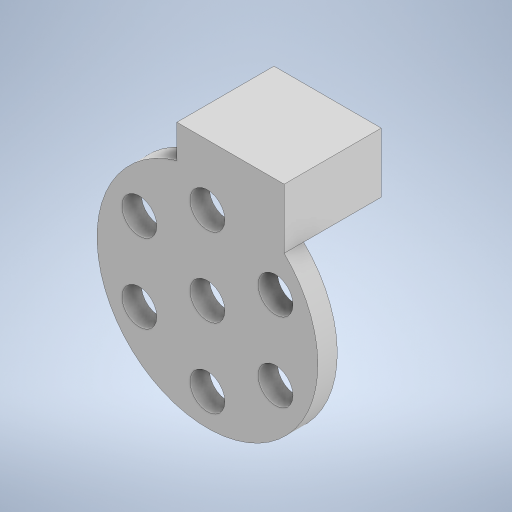
# Autodesk Inventor part: revolver
Saved by Autodesk Inventor 2023.1 (Build 271208000, 208)
## iProperties
Created: 2023-04-12
Part Number: revolver
Material: Типовые
Document SubType Name: Modeling
Designer: User
Density: 1 g/cm^3
Appearance: По умолчанию
Author: User
Autodesk Inventor part; units mm, degrees
(part 1 of 8)
ref_plane "YZ Plane" through (0, 0, 0) normal (1, 0, 0) x (0, 1, 0)
ref_plane "XZ Plane" through (0, 0, 0) normal (0, 1, 0) x (-1, 0, 0)
ref_plane "XY Plane" through (0, 0, 0) normal (0, 0, 1) x (1, 0, 0)
sketch "Эскиз1" plane through (0, 0, 0) normal (0, 0, 1) x (1, 0, 0)
  line L0 (-22.838, -17.5712) -> (24.4153, -17.5965)
  arc A0 (24.4153, -17.5965) -> (25.2491, -16.7631) centre (24.4158, -16.7631) ccw
  line L1 (25.2491, -16.7631) -> (25.2491, 45.1296)
  arc A1 (25.2491, 45.1296) -> (24.4158, 45.963) centre (24.4158, 45.1296) ccw
  line L2 (24.4158, 45.963) -> (-5.7821, 45.963)
  line L3 (-5.7821, 45.963) -> (-5.7821, 46.7963)
  line L4 (-5.7821, 46.7963) -> (24.4158, 46.7963)
  arc A2 (26.0825, 45.1296) -> (24.4158, 46.7963) centre (24.4158, 45.1296) ccw
  line L5 (26.0825, 45.1296) -> (26.0825, -16.7631)
  arc A3 (24.4149, -18.4298) -> (26.0825, -16.7631) centre (24.4158, -16.7631) ccw
  line L6 (24.4149, -18.4298) -> (-22.851, -18.4045)
  arc A4 (-24.5167, -16.7369) -> (-22.851, -18.4045) centre (-22.8501, -16.7378) ccw
  line L7 (-24.5167, -16.7369) -> (-24.5023, 10.1628)
  line L8 (-24.5023, 10.1628) -> (-24.5023, 45.1296)
  arc A5 (-22.8357, 46.7963) -> (-24.5023, 45.1296) centre (-22.8357, 45.1296) ccw
  line L9 (-22.8357, 46.7963) -> (-21.4453, 46.7963)
  line L10 (-21.4453, 46.7963) -> (-21.4453, 45.9649)
  line L11 (-21.4453, 45.9649) -> (-22.8357, 45.9649)
  arc A6 (-22.8357, 45.9649) -> (-23.6709, 45.1296) centre (-22.8357, 45.1296) ccw
  line L12 (-23.6709, 45.1296) -> (-23.6709, -16.7378)
  arc A7 (-23.6709, -16.7378) -> (-22.838, -17.5712) centre (-22.8376, -16.7378) ccw
  arc A8 (-21.1689, 72.3508) -> (-19.5022, 70.6842) centre (-19.5022, 72.3508) ccw
  line L13 (-21.1689, 72.3508) -> (-21.1689, 75.1651)
  arc A9 (-19.5022, 76.8318) -> (-21.1689, 75.1651) centre (-19.5022, 75.1651) ccw
  line L14 (-19.5022, 76.8318) -> (21.0482, 76.8318)
  arc A10 (22.7149, 75.1651) -> (21.0482, 76.8318) centre (21.0482, 75.1651) ccw
  line L15 (22.7149, 75.1651) -> (22.7149, 72.3508)
  arc A11 (21.0482, 70.6842) -> (22.7149, 72.3508) centre (21.0482, 72.3508) ccw
  line L16 (21.0482, 70.6842) -> (-19.5022, 70.6842)
  arc A12 (-21.1685, 54.6279) -> (-19.5018, 52.9613) centre (-19.5018, 54.6279) ccw
  line L17 (-21.1685, 54.6279) -> (-21.1685, 67.6609)
  arc A13 (-19.5018, 69.3275) -> (-21.1685, 67.6609) centre (-19.5018, 67.6609) ccw
  line L18 (-19.5018, 69.3275) -> (21.0483, 69.3275)
  arc A14 (22.715, 67.6609) -> (21.0483, 69.3275) centre (21.0483, 67.6609) ccw
  line L19 (22.715, 67.6609) -> (22.715, 54.6279)
  arc A15 (21.0483, 52.9613) -> (22.715, 54.6279) centre (21.0483, 54.6279) ccw
  line L20 (21.0483, 52.9613) -> (-19.5018, 52.9613)
  line L21 (19.3067, -63.6373) -> (19.3067, -61.3545)
  line L22 (19.3067, -61.3545) -> (18.828, -61.3545)
  line L23 (18.828, -61.3545) -> (18.0508, -63.7032)
  line L24 (7.2647, -61.3545) -> (6.4355, -61.3545)
  line L25 (6.4355, -61.3545) -> (6.4355, -63.6373)
  line L26 (4.7702, -63.0128) -> (4.7702, -61.3545)
  line L27 (4.7702, -61.3545) -> (3.9411, -61.3545)
  line L28 (-4.7774, -61.1463) -> (-4.7774, -62.1837)
  line L29 (-4.7774, -62.1837) -> (-3.5353, -62.1837)
  line L30 (-3.5353, -62.1837) -> (-3.5353, -61.1463)
  line L31 (-3.5353, -63.6373) -> (-3.5353, -62.6)
  line L32 (-3.5353, -62.6) -> (-4.7774, -62.6)
  line L33 (-4.7774, -62.6) -> (-4.7774, -63.6373)
  line L34 (-13.5409, -61.1463) -> (-13.5409, -62.371)
  line L35 (-13.5409, -62.371) -> (-12.2225, -60.9868)
  line L36 (-11.9485, -61.3025) -> (-12.7846, -62.1802)
  line L37 (-12.7846, -62.1802) -> (-11.9276, -63.502)
  line L38 (-15.1645, -63.0128) -> (-15.1645, -61.3545)
  line L39 (-15.1645, -61.3545) -> (-15.9937, -61.3545)
  line L40 (-10.0766, -55.8058) -> (-10.8765, -54.608)
  line L41 (-10.8765, -54.608) -> (-11.6765, -55.8058)
  line L42 (-12.104, -55.5222) -> (-11.1855, -54.1466)
  line L43 (-11.1855, -54.1466) -> (-12.104, -52.771)
  line L44 (-11.6765, -52.4875) -> (-10.8765, -53.6853)
  line L45 (-10.8765, -53.6853) -> (-10.0766, -52.4875)
  line L46 (-9.6491, -52.771) -> (-10.5676, -54.1466)
  line L47 (-10.5676, -54.1466) -> (-9.6491, -55.5222)
  line L48 (-20.3629, -49.5032) -> (-18.6809, -54.4768)
  line L49 (-18.6809, -54.4768) -> (-16.999, -49.5032)
  line L50 (14.3835, -41.5364) -> (15.2126, -41.5364)
  line L51 (15.2126, -41.5364) -> (15.2126, -40.7072)
  line L52 (15.2126, -40.7072) -> (14.3835, -40.7072)
  line L53 (15.2126, -42.99) -> (15.2126, -41.9527)
  line L54 (15.2126, -41.9527) -> (14.7026, -41.9527)
  line L55 (14.7026, -41.9527) -> (13.9359, -43.1045)
  line L56 (12.3053, -42.3655) -> (12.3053, -40.7072)
  line L57 (12.3053, -40.7072) -> (11.4762, -40.7072)
  line L58 (-0.9857, -42.99) -> (-0.9857, -40.7072)
  line L59 (-0.9857, -40.7072) -> (-1.4645, -40.7072)
  line L60 (-1.4645, -40.7072) -> (-2.2416, -43.0559)
  line L61 (-13.0277, -40.7072) -> (-13.8569, -40.7072)
  line L62 (-13.8569, -40.7072) -> (-13.8569, -42.99)
  line L63 (-15.5222, -42.3655) -> (-15.5222, -40.7072)
  line L64 (-15.5222, -40.7072) -> (-16.3514, -40.7072)
  line L65 (20.5386, -19.6576) -> (19.7094, -19.6576)
  line L66 (19.7094, -19.6576) -> (19.7094, -21.7323)
  line L67 (19.7094, -21.7323) -> (20.5386, -21.7323)
  line L68 (20.5386, -22.1486) -> (19.7094, -22.1486)
  line L69 (19.7094, -22.1486) -> (19.7094, -23.186)
  line L70 (16.8021, -20.0705) -> (16.8021, -20.4868)
  line L71 (16.8021, -20.4868) -> (18.0442, -20.4868)
  line L72 (18.0442, -20.4868) -> (18.0442, -20.0705)
  line L73 (18.2523, -20.9031) -> (16.8021, -20.9031)
  line L74 (16.8021, -20.9031) -> (16.8021, -21.316)
  line L75 (-18.1801, -30.8646) -> (-18.1801, -34.3929)
  line L76 (-18.1801, -34.3929) -> (-16.7265, -34.3929)
  line L77 (-6.2745, -20.9508) -> (-7.1037, -20.9508)
  line L78 (-7.1037, -20.9508) -> (-7.1037, -21.78)
  line L79 (-7.1037, -21.78) -> (-6.2745, -21.78)
  line L80 (-7.1037, -19.4972) -> (-7.1037, -20.5345)
  line L81 (-7.1037, -20.5345) -> (-6.2745, -20.5345)
  line L82 (-12.0891, -21.78) -> (-11.26, -21.78)
  line L83 (-11.26, -21.78) -> (-11.26, -19.4972)
  line L84 (8.677, -7.6777) -> (7.8478, -7.6777)
  line L85 (7.8478, -7.6777) -> (7.8478, -9.9605)
  line L86 (6.1825, -9.336) -> (6.1825, -7.6777)
  line L87 (6.1825, -7.6777) -> (5.3534, -7.6777)
  line L88 (6.8528, 0.8169) -> (6.0236, 0.8169)
  line L89 (6.0236, 0.8169) -> (6.0236, -1.4659)
  line L90 (-11.1301, -10.0439) -> (-11.1301, -9.2147)
  line L91 (-11.1301, -9.2147) -> (-12.3756, -9.2147)
  line L92 (-12.3722, -8.7984) -> (-11.1301, -8.7984)
  line L93 (-11.1301, -8.7984) -> (-11.1301, -6.9319)
  line L94 (-17.146, -7.1401) -> (-18.6031, -7.1401)
  line L95 (-18.6031, -7.1401) -> (-18.6031, -8.3856)
  line L96 (-18.6031, -8.3856) -> (-17.5588, -8.3856)
  line L97 (-17.5588, -8.8019) -> (-18.6031, -8.8019)
  line L98 (-18.6031, -8.8019) -> (-18.6031, -10.4602)
  line L99 (-18.6031, -10.4602) -> (-17.146, -10.4602)
  line L100 (-8.8573, 0.7006) -> (-9.6865, 0.7006)
  line L101 (-9.6865, 0.7006) -> (-9.6865, -1.3741)
  line L102 (-9.6865, -1.3741) -> (-8.8573, -1.3741)
  line L103 (-8.8573, -1.7904) -> (-9.6865, -1.7904)
  line L104 (-9.6865, -1.7904) -> (-9.6865, -2.8277)
  line L105 (-18.4084, 0.9087) -> (-18.4084, -0.1286)
  line L106 (-18.4084, -0.1286) -> (-17.1664, -0.1286)
  line L107 (-17.1664, -0.1286) -> (-17.1664, 0.9087)
  line L108 (-17.1664, -1.5823) -> (-17.1664, -0.5449)
  line L109 (-17.1664, -0.5449) -> (-18.4084, -0.5449)
  line L110 (-18.4084, -0.5449) -> (-18.4084, -1.5823)
  line L111 (17.3177, 22.7837) -> (17.3177, 24.5136)
  line L112 (17.3177, 24.5136) -> (16.7676, 24.5136)
  line L113 (16.7676, 24.5136) -> (16.7676, 22.7837)
  line L114 (18.0107, 24.5136) -> (17.7357, 24.5136)
  line L115 (17.7357, 24.5136) -> (17.7357, 22.7837)
  line L116 (12.8402, 24.5136) -> (12.2407, 24.5136)
  line L117 (12.2407, 24.5136) -> (12.2407, 22.7837)
  line L118 (-7.5678, 13.3431) -> (-7.5678, 16.3093)
  line L119 (-7.5678, 16.3093) -> (-8.4247, 14.873)
  line L120 (-8.782, 14.873) -> (-9.6459, 16.3093)
  line L121 (-9.6459, 16.3093) -> (-9.6459, 13.3431)
  line L122 (-9.6737, 17.1697) -> (-8.6051, 15.3865)
  line L123 (-8.6051, 15.3865) -> (-7.54, 17.1697)
  line L124 (-15.6721, 13.5512) -> (-14.6348, 13.5512)
  line L125 (-14.6348, 13.5512) -> (-14.6348, 15.2096)
  line L126 (-14.6348, 15.2096) -> (-14.8395, 15.2096)
  line L127 (-15.6588, 18.5916) -> (-14.6215, 18.5916)
  line L128 (-14.6215, 18.5916) -> (-14.6215, 20.2499)
  line L129 (-14.6215, 20.2499) -> (-14.8262, 20.2499)
  line L130 (-14.5012, 31.7916) -> (-13.0071, 31.7916)
  line L131 (-13.0071, 31.7916) -> (-13.7521, 34.0264)
  line L132 (-13.7521, 34.0264) -> (-14.5012, 31.7916)
  line L133 (-12.4696, 30.179) -> (-12.8336, 31.2752)
  line L134 (-12.8336, 31.2752) -> (-14.6748, 31.2752)
  line L135 (-14.6748, 31.2752) -> (-15.0388, 30.179)
  line L136 (-18.0947, 32.5323) -> (-19.1063, 32.5323)
  line L137 (-19.1063, 32.5323) -> (-19.1063, 30.5091)
  line L138 (-19.1063, 30.5091) -> (-18.0947, 30.5091)
  line L139 (-17.0831, 34.5597) -> (-19.1063, 34.5597)
  line L140 (-19.1063, 34.5597) -> (-19.1063, 33.0402)
  line L141 (-19.1063, 33.0402) -> (-18.0947, 33.0402)
  line L142 (12.3369, 89.0704) -> (15.2204, 89.0704)
  line L143 (15.2204, 89.0704) -> (15.2204, 84.693)
  line L144 (15.2204, 84.693) -> (14.483, 84.693)
  line L145 (14.483, 84.693) -> (14.483, 88.4511)
  line L146 (14.483, 88.4511) -> (12.9798, 88.4511)
  line L147 (11.3583, 84.693) -> (11.3583, 85.3359)
  line L148 (11.3583, 85.3359) -> (11.3961, 85.3359)
  line L149 (3.7854, 84.9152) -> (3.7854, 83.0811)
  line L150 (3.7854, 83.0811) -> (3.048, 83.0811)
  line L151 (3.048, 83.0811) -> (3.048, 89.0704)
  line L152 (3.048, 89.0704) -> (3.7854, 89.0704)
  line L153 (3.7854, 89.0704) -> (3.7854, 88.6119)
  line L154 (-2.497, 84.693) -> (-2.497, 86.6643)
  line L155 (-2.497, 86.6643) -> (-4.473, 86.6643)
  line L156 (-4.473, 86.6643) -> (-4.473, 84.693)
  line L157 (-4.473, 84.693) -> (-5.2104, 84.693)
  line L158 (-5.2104, 84.693) -> (-5.2104, 89.0704)
  line L159 (-5.2104, 89.0704) -> (-4.473, 89.0704)
  line L160 (-4.473, 89.0704) -> (-4.473, 87.2977)
  line L161 (-4.473, 87.2977) -> (-2.497, 87.2977)
  line L162 (-2.497, 87.2977) -> (-2.497, 89.0704)
  line L163 (-2.497, 89.0704) -> (-1.7596, 89.0704)
  line L164 (-1.7596, 89.0704) -> (-1.7596, 84.693)
  line L165 (-1.7596, 84.693) -> (-2.497, 84.693)
  line L166 (-1.6305, 80.6448) -> (-2.0468, 80.6448)
  line L167 (-2.0468, 80.6448) -> (-2.0468, 79.8157)
  line L168 (-2.0468, 79.8157) -> (-1.6305, 79.8157)
  line L169 (-2.0468, 82.0985) -> (-2.0468, 81.0612)
  line L170 (-2.0468, 81.0612) -> (-1.6305, 81.0612)
  line L171 (-11.1885, 79.6075) -> (-11.1885, 81.8903)
  line L172 (-11.1885, 81.8903) -> (-12.0177, 81.8903)
  line L173 (-12.0177, 81.8903) -> (-12.0177, 79.6075)
  line L174 (-10.3559, 81.8903) -> (-10.7722, 81.8903)
  line L175 (-10.7722, 81.8903) -> (-10.7722, 79.6075)
  line L176 (-17.0031, 79.8157) -> (-16.174, 79.8157)
  line L177 (-16.174, 79.8157) -> (-16.174, 82.0985)
  arc A16 (-22.8351, -20.4439) -> (-24.5018, -22.1106) centre (-22.8351, -22.1106) ccw
  line L178 (-22.8351, -20.4439) -> (-21.4448, -20.4439)
  line L179 (-21.4448, -20.4439) -> (-21.4448, -21.2772)
  line L180 (-21.4448, -21.2772) -> (-22.8351, -21.2772)
  arc A17 (-22.8351, -21.2772) -> (-23.6685, -22.1106) centre (-22.8351, -22.1106) ccw
  line L181 (-23.6685, -22.1106) -> (-23.6685, -35.3124)
  arc A18 (-23.6685, -35.3124) -> (-22.8351, -36.1457) centre (-22.8351, -35.3124) ccw
  line L182 (-22.8351, -36.1457) -> (-0.1596, -36.1457)
  arc A19 (-0.1596, -36.1457) -> (0.6737, -35.3124) centre (-0.1596, -35.3124) ccw
  line L183 (0.6737, -35.3124) -> (0.6737, -22.1106)
  arc A20 (0.6737, -22.1106) -> (-0.1596, -21.2772) centre (-0.1596, -22.1106) ccw
  line L184 (-0.1596, -21.2772) -> (-2.846, -21.2772)
  line L185 (-2.846, -21.2772) -> (-2.846, -20.4439)
  line L186 (-2.846, -20.4439) -> (-0.1596, -20.4439)
  arc A21 (1.5071, -22.1106) -> (-0.1596, -20.4439) centre (-0.1596, -22.1106) ccw
  line L187 (1.5071, -22.1106) -> (1.5071, -35.3124)
  arc A22 (-0.1596, -36.9791) -> (1.5071, -35.3124) centre (-0.1596, -35.3124) ccw
  line L188 (-0.1596, -36.9791) -> (-22.8351, -36.9791)
  arc A23 (-24.5018, -35.3124) -> (-22.8351, -36.9791) centre (-22.8351, -35.3124) ccw
  line L189 (-24.5018, -35.3124) -> (-24.5018, -22.1106)
  line L190 (5.6148, -20.4439) -> (5.6148, -21.2772)
  line L191 (5.6148, -21.2772) -> (4.9165, -21.2772)
  arc A24 (4.9165, -21.2772) -> (4.0832, -22.1106) centre (4.9165, -22.1106) ccw
  line L192 (4.0832, -22.1106) -> (4.0832, -35.3124)
  arc A25 (4.0832, -35.3124) -> (4.9165, -36.1457) centre (4.9165, -35.3124) ccw
  line L193 (4.9165, -36.1457) -> (24.3817, -36.1457)
  arc A26 (24.3817, -36.1457) -> (25.215, -35.3124) centre (24.3817, -35.3124) ccw
  line L194 (25.215, -35.3124) -> (25.215, -22.1106)
  arc A27 (25.215, -22.1106) -> (24.3817, -21.2772) centre (24.3817, -22.1106) ccw
  line L195 (24.3817, -21.2772) -> (23.3418, -21.2772)
  line L196 (23.3418, -21.2772) -> (23.3418, -20.4439)
  line L197 (23.3418, -20.4439) -> (24.3817, -20.4439)
  arc A28 (26.0483, -22.1106) -> (24.3817, -20.4439) centre (24.3817, -22.1106) ccw
  line L198 (26.0483, -22.1106) -> (26.0483, -35.3124)
  arc A29 (24.3817, -36.9791) -> (26.0483, -35.3124) centre (24.3817, -35.3124) ccw
  line L199 (24.3817, -36.9791) -> (4.9165, -36.9791)
  arc A30 (3.2498, -35.3124) -> (4.9165, -36.9791) centre (4.9165, -35.3124) ccw
  line L200 (3.2498, -35.3124) -> (3.2498, -22.1106)
  arc A31 (4.9165, -20.4439) -> (3.2498, -22.1106) centre (4.9165, -22.1106) ccw
  line L201 (4.9165, -20.4439) -> (5.6148, -20.4439)
  arc A32 (-22.9167, -41.4487) -> (-24.5833, -43.1153) centre (-22.9167, -43.1153) ccw
  line L202 (-22.9167, -41.4487) -> (-21.4448, -41.4487)
  line L203 (-21.4448, -41.4487) -> (-21.4448, -42.282)
  line L204 (-21.4448, -42.282) -> (-22.9167, -42.282)
  arc A33 (-22.9167, -42.282) -> (-23.75, -43.1153) centre (-22.9167, -43.1153) ccw
  line L205 (-23.75, -43.1153) -> (-23.75, -85.5941)
  arc A34 (-23.75, -85.5941) -> (-22.9167, -86.4275) centre (-22.9167, -85.5941) ccw
  line L206 (-22.9167, -86.4275) -> (24.1667, -86.4275)
  arc A35 (24.1667, -86.4275) -> (25, -85.5941) centre (24.1667, -85.5941) ccw
  line L207 (25, -85.5941) -> (25, -43.1153)
  arc A36 (25, -43.1153) -> (24.1667, -42.282) centre (24.1667, -43.1153) ccw
  line L208 (24.1667, -42.282) -> (17.2706, -42.282)
  line L209 (17.2706, -42.282) -> (17.2706, -41.4487)
  line L210 (17.2706, -41.4487) -> (24.1667, -41.4487)
  arc A37 (25.8333, -43.1153) -> (24.1667, -41.4487) centre (24.1667, -43.1153) ccw
  line L211 (25.8333, -43.1153) -> (25.8333, -85.5941)
  arc A38 (24.1667, -87.2608) -> (25.8333, -85.5941) centre (24.1667, -85.5941) ccw
  line L212 (24.1667, -87.2608) -> (-22.9167, -87.2608)
  arc A39 (-24.5833, -85.5941) -> (-22.9167, -87.2608) centre (-22.9167, -85.5941) ccw
  line L213 (-24.5833, -85.5941) -> (-24.5833, -43.1153)
  line L214 (-8.2778, 81.4775) -> (-8.2778, 81.0612)
  line L215 (-8.2778, 81.0612) -> (-7.0357, 81.0612)
  line L216 (-7.0357, 81.0612) -> (-7.0357, 81.4775)
  line L217 (-6.8276, 80.6448) -> (-8.2778, 80.6448)
  line L218 (-8.2778, 80.6448) -> (-8.2778, 80.232)
  line L219 (-3.7121, 79.6075) -> (-3.7121, 81.4532)
  line L220 (-3.7121, 81.4532) -> (-4.3713, 80.5269)
  line L221 (-4.7113, 80.5269) -> (-5.3705, 81.4532)
  line L222 (-5.3705, 81.4532) -> (-5.3705, 79.6075)
  line L223 (-5.4086, 82.2199) -> (-4.5413, 81.0022)
  line L224 (-4.5413, 81.0022) -> (-3.674, 82.2199)
  line L225 (-11.819, 87.0188) -> (-10.0416, 84.693)
  line L226 (-10.0416, 84.693) -> (-10.9587, 84.693)
  line L227 (-10.9587, 84.693) -> (-12.4572, 86.7115)
  line L228 (-12.4572, 86.7115) -> (-12.8212, 86.7115)
  line L229 (-12.8212, 86.7115) -> (-12.8212, 84.693)
  line L230 (-12.8212, 84.693) -> (-13.5586, 84.693)
  line L231 (-13.5586, 84.693) -> (-13.5586, 89.0704)
  line L232 (-13.5586, 89.0704) -> (-12.8212, 89.0704)
  line L233 (-12.8212, 89.0704) -> (-12.8212, 87.1653)
  line L234 (-10.5427, 89.0704) -> (-10.3441, 89.0704)
  line L235 (-10.3441, 89.0704) -> (-10.3441, 88.4369)
  line L236 (-10.3441, 88.4369) -> (-10.5143, 88.4369)
  line L237 (1.0105, 88.4275) -> (1.0105, 84.693)
  line L238 (1.0105, 84.693) -> (0.2731, 84.693)
  line L239 (0.2731, 84.693) -> (0.2731, 88.4275)
  line L240 (0.2731, 88.4275) -> (-1.216, 88.4275)
  line L241 (-1.216, 88.4275) -> (-1.216, 89.0704)
  line L242 (-1.216, 89.0704) -> (2.4996, 89.0704)
  line L243 (2.4996, 89.0704) -> (2.4996, 88.4275)
  line L244 (2.4996, 88.4275) -> (1.0105, 88.4275)
  line L245 (17.5746, 86.7683) -> (17.0262, 86.7683)
  line L246 (17.0262, 86.7683) -> (17.0262, 85.2792)
  line L247 (17.0262, 85.2792) -> (17.5557, 85.2792)
  line L248 (17.8204, 84.693) -> (16.2888, 84.693)
  line L249 (16.2888, 84.693) -> (16.2888, 89.0704)
  line L250 (16.2888, 89.0704) -> (17.0262, 89.0704)
  line L251 (17.0262, 89.0704) -> (17.0262, 87.3639)
  line L252 (17.0262, 87.3639) -> (17.8393, 87.3639)
  line L253 (-16.8523, 43.0002) -> (-17.6815, 43.0002)
  line L254 (-17.6815, 43.0002) -> (-17.6815, 41.3419)
  line L255 (-17.6815, 41.3419) -> (-16.8523, 41.3419)
  line L256 (-16.8523, 40.9256) -> (-17.6815, 40.9256)
  line L257 (-17.6815, 40.9256) -> (-17.6815, 39.4719)
  line L258 (-14.3579, 43.2084) -> (-14.3579, 41.7548)
  line L259 (-14.3579, 41.7548) -> (-12.6996, 41.7548)
  line L260 (-12.6996, 41.7548) -> (-12.6996, 43.2188)
  line L261 (-12.6996, 39.4719) -> (-12.6996, 41.3384)
  line L262 (-12.6996, 41.3384) -> (-14.3579, 41.3384)
  line L263 (-14.3579, 41.3384) -> (-14.3579, 39.4719)
  line L264 (-4.9187, 31.017) -> (-4.9187, 32.0286)
  line L265 (-4.9187, 32.0286) -> (-6.4382, 32.0286)
  line L266 (-6.4339, 32.5365) -> (-4.9187, 32.5365)
  line L267 (-4.9187, 32.5365) -> (-4.9187, 34.8136)
  line L268 (-12.1271, 21.9117) -> (-12.9562, 21.9117)
  line L269 (-12.9562, 21.9117) -> (-12.9562, 20.2534)
  line L270 (-12.9562, 20.2534) -> (-12.1271, 20.2534)
  line L271 (-12.1271, 19.837) -> (-12.9562, 19.837)
  line L272 (-12.9562, 19.837) -> (-12.9562, 18.3834)
  line L273 (-2.041, 24.5306) -> (-2.6405, 24.5306)
  line L274 (-2.6405, 24.5306) -> (-2.6405, 23.007)
  line L275 (-2.6405, 23.007) -> (-2.041, 23.007)
  line L276 (-2.041, 22.5917) -> (-2.6405, 22.5917)
  line L277 (-2.6405, 22.5917) -> (-2.6405, 21.8326)
  line L278 (0.5003, 23.2848) -> (0.5003, 24.5306)
  line L279 (0.5003, 24.5306) -> (-0.102, 24.5306)
  line L280 (2.1614, 24.9459) -> (2.2412, 24.9459)
  line L281 (2.2412, 24.9459) -> (1.5289, 25.5565)
  line L282 (2.97, 25.4987) -> (2.1312, 25.4987)
  line L283 (2.1312, 25.4987) -> (2.97, 24.7644)
  line L284 (15.3815, 22.2997) -> (15.3815, 22.5747)
  line L285 (15.3815, 22.5747) -> (14.7819, 22.5747)
  line L286 (14.7792, 22.99) -> (15.3815, 22.99)
  line L287 (15.3815, 22.99) -> (15.3815, 24.7199)
  line L288 (-14.2591, -0.9578) -> (-14.2591, 0.7006)
  line L289 (-14.2591, 0.7006) -> (-15.0883, 0.7006)
  line L290 (-11.7646, 0.7006) -> (-12.5938, 0.7006)
  line L291 (-12.5938, 0.7006) -> (-12.5938, -1.5823)
  line L292 (-13.2735, 3.7618) -> (-14.4913, 5.9301)
  line L293 (-14.4913, 5.9301) -> (-14.9839, 5.4444)
  line L294 (-14.9839, 5.4444) -> (-14.9839, 3.8624)
  line L295 (-14.9839, 7.5989) -> (-14.9839, 6.0099)
  line L296 (-14.9839, 6.0099) -> (-13.2354, 7.7446)
  line L297 (-12.9439, 7.4531) -> (-14.1825, 6.2215)
  line L298 (-14.1825, 6.2215) -> (-12.9058, 3.963)
  line L299 (-7.8065, -10.6684) -> (-7.8065, -7.1401)
  line L300 (-7.8065, -7.1401) -> (-9.4649, -7.1401)
  line L301 (-9.4649, -7.1401) -> (-9.4649, -10.6684)
  line L302 (10.1729, -0.8414) -> (10.1729, 0.8169)
  line L303 (10.1729, 0.8169) -> (9.3438, 0.8169)
  line L304 (12.6674, 0.8169) -> (11.8382, 0.8169)
  line L305 (11.8382, 0.8169) -> (11.8382, -1.2577)
  line L306 (11.8382, -1.2577) -> (12.6674, -1.2577)
  line L307 (12.6674, -1.674) -> (11.8382, -1.674)
  line L308 (11.8382, -1.674) -> (11.8382, -2.7114)
  line L309 (11.9971, -9.336) -> (11.9971, -7.6777)
  line L310 (11.9971, -7.6777) -> (11.168, -7.6777)
  line L311 (14.9044, -9.9605) -> (14.9044, -7.6777)
  line L312 (14.9044, -7.6777) -> (14.4257, -7.6777)
  line L313 (14.4257, -7.6777) -> (13.6485, -10.0264)
  line L314 (-17.0746, -21.3637) -> (-17.0746, -19.7053)
  line L315 (-17.0746, -19.7053) -> (-17.9037, -19.7053)
  line L316 (-14.5801, -19.7053) -> (-15.4093, -19.7053)
  line L317 (-15.4093, -19.7053) -> (-15.4093, -21.9882)
  line L318 (-17.474, -25.5939) -> (-18.5114, -25.5939)
  line L319 (-18.5114, -25.5939) -> (-18.5114, -28.914)
  line L320 (-18.5114, -28.914) -> (-17.474, -28.914)
  line L321 (-19.6338, -31.0727) -> (-21.0874, -31.0727)
  line L322 (-21.0874, -31.0727) -> (-21.0874, -32.3113)
  line L323 (-21.0874, -32.3113) -> (-19.6338, -32.3113)
  line L324 (-19.6338, -32.7276) -> (-21.0874, -32.7276)
  line L325 (-21.0874, -32.7276) -> (-21.0874, -34.601)
  line L326 (8.2849, -21.7323) -> (9.1141, -21.7323)
  line L327 (9.1141, -21.7323) -> (9.1141, -19.4495)
  line L328 (15.1369, -21.9405) -> (15.1369, -20.0948)
  line L329 (15.1369, -20.0948) -> (14.4777, -21.0211)
  line L330 (14.1377, -21.0211) -> (13.4785, -20.0948)
  line L331 (13.4785, -20.0948) -> (13.4785, -21.9405)
  line L332 (13.4404, -19.3281) -> (14.3077, -20.5458)
  line L333 (14.3077, -20.5458) -> (15.175, -19.3281)
  line L334 (6.2997, -24.2855) -> (6.4627, -24.2855)
  line L335 (6.4627, -24.2855) -> (5.5329, -23.3973)
  line L336 (7.337, -23.4563) -> (6.1956, -23.4563)
  line L337 (6.1956, -23.4563) -> (7.2954, -24.5075)
  line L338 (10.0361, -26.3601) -> (10.0361, -24.7018)
  line L339 (10.0361, -24.7018) -> (9.207, -24.7018)
  line L340 (12.5306, -24.7018) -> (11.7014, -24.7018)
  line L341 (11.7014, -24.7018) -> (11.7014, -26.7765)
  line L342 (11.7014, -26.7765) -> (12.5306, -26.7765)
  line L343 (12.5306, -27.1928) -> (11.7014, -27.1928)
  line L344 (11.7014, -27.1928) -> (11.7014, -28.2301)
  line L345 (7.0741, -32.5952) -> (7.0741, -30.9369)
  line L346 (7.0741, -30.9369) -> (6.245, -30.9369)
  line L347 (8.6978, -30.7287) -> (8.6978, -31.9534)
  line L348 (8.6978, -31.9534) -> (10.0161, -30.5691)
  line L349 (10.2902, -30.8848) -> (9.4541, -31.7626)
  line L350 (9.4541, -31.7626) -> (10.311, -33.0844)
  line L351 (-19.6715, -40.499) -> (-19.6715, -41.5364)
  line L352 (-19.6715, -41.5364) -> (-18.4295, -41.5364)
  line L353 (-18.4295, -41.5364) -> (-18.4295, -40.499)
  line L354 (-18.4295, -42.99) -> (-18.4295, -41.9527)
  line L355 (-18.4295, -41.9527) -> (-19.6715, -41.9527)
  line L356 (-19.6715, -41.9527) -> (-19.6715, -42.99)
  line L357 (-10.1204, -40.7072) -> (-10.9496, -40.7072)
  line L358 (-10.9496, -40.7072) -> (-10.9496, -42.7819)
  line L359 (-10.9496, -42.7819) -> (-10.1204, -42.7819)
  line L360 (-10.1204, -43.1982) -> (-10.9496, -43.1982)
  line L361 (-10.9496, -43.1982) -> (-10.9496, -44.2355)
  line L362 (-6.8003, -42.3655) -> (-6.8003, -40.7072)
  line L363 (-6.8003, -40.7072) -> (-7.6295, -40.7072)
  line L364 (1.0924, -41.5364) -> (1.9216, -41.5364)
  line L365 (1.9216, -41.5364) -> (1.9216, -40.7072)
  line L366 (1.9216, -40.7072) -> (1.0924, -40.7072)
  line L367 (1.9216, -42.99) -> (1.9216, -41.9527)
  line L368 (1.9216, -41.9527) -> (1.4116, -41.9527)
  line L369 (1.4116, -41.9527) -> (0.6449, -43.1045)
  line L370 (3.5869, -40.499) -> (3.5869, -41.5364)
  line L371 (3.5869, -41.5364) -> (3.9997, -41.5364)
  line L372 (3.9997, -41.5364) -> (3.9997, -40.9952)
  line L373 (3.9997, -42.4939) -> (3.9997, -41.9527)
  line L374 (3.9997, -41.9527) -> (3.5869, -41.9527)
  line L375 (3.5869, -41.9527) -> (3.5869, -42.99)
  line L376 (8.156, -40.499) -> (8.156, -42.7819)
  line L377 (8.156, -42.7819) -> (8.9852, -42.7819)
  line L378 (8.9852, -42.7819) -> (8.9852, -40.499)
  line L379 (9.4015, -40.499) -> (9.4015, -42.7819)
  line L380 (9.4015, -42.7819) -> (9.6097, -42.7819)
  line L381 (9.4015, -43.4029) -> (9.4015, -43.1982)
  line L382 (9.4015, -43.1982) -> (7.3234, -43.1982)
  line L383 (7.3268, -42.7819) -> (7.7397, -42.7819)
  line L384 (7.7397, -42.7819) -> (7.7397, -40.499)
  line L385 (-19.3139, -61.1463) -> (-19.3139, -62.1837)
  line L386 (-19.3139, -62.1837) -> (-18.0718, -62.1837)
  line L387 (-18.0718, -62.1837) -> (-18.0718, -61.1463)
  line L388 (-18.0718, -63.6373) -> (-18.0718, -62.6)
  line L389 (-18.0718, -62.6) -> (-19.3139, -62.6)
  line L390 (-19.3139, -62.6) -> (-19.3139, -63.6373)
  line L391 (-9.3499, -63.6373) -> (-9.3499, -61.3545)
  line L392 (-9.3499, -61.3545) -> (-9.8287, -61.3545)
  line L393 (-9.8287, -61.3545) -> (-10.6058, -63.7032)
  line L394 (0.6209, -61.1463) -> (0.6209, -62.1837)
  line L395 (0.6209, -62.1837) -> (1.8629, -62.1837)
  line L396 (1.8629, -62.1837) -> (1.8629, -61.1463)
  line L397 (1.8629, -63.6373) -> (1.8629, -62.6)
  line L398 (1.8629, -62.6) -> (0.6209, -62.6)
  line L399 (0.6209, -62.6) -> (0.6209, -63.6373)
  line L400 (10.172, -61.3545) -> (9.3428, -61.3545)
  line L401 (9.3428, -61.3545) -> (9.3428, -63.4292)
  line L402 (9.3428, -63.4292) -> (10.172, -63.4292)
  line L403 (10.172, -63.8455) -> (9.3428, -63.8455)
  line L404 (9.3428, -63.8455) -> (9.3428, -64.8828)
  line L405 (13.4921, -63.0128) -> (13.4921, -61.3545)
  line L406 (13.4921, -61.3545) -> (12.663, -61.3545)
  line L407 (-8.0227, 46.4791) -> (-8.8519, 46.4791)
  line L408 (-8.8519, 46.4791) -> (-8.8519, 45.6499)
  line L409 (-8.8519, 45.6499) -> (-8.0227, 45.6499)
  line L410 (-8.8519, 47.9327) -> (-8.8519, 46.8954)
  line L411 (-8.8519, 46.8954) -> (-8.0227, 46.8954)
  arc A40 (-22.8357, 81.354) -> (-24.5023, 79.6873) centre (-22.8357, 79.6873) ccw
  line L412 (-22.8357, 81.354) -> (-21.4453, 81.354)
  line L413 (-21.4453, 81.354) -> (-21.4453, 80.5205)
  line L414 (-21.4453, 80.5205) -> (-22.8357, 80.5205)
  arc A41 (-22.8357, 80.5205) -> (-23.6689, 79.6873) centre (-22.8357, 79.6873) ccw
  line L415 (-23.6689, 79.6873) -> (-23.6689, 52.1086)
  arc A42 (-23.6689, 52.1086) -> (-22.8357, 51.2754) centre (-22.8357, 52.1086) ccw
  line L416 (-22.8357, 51.2754) -> (24.3817, 51.2754)
  arc A43 (24.3817, 51.2754) -> (25.2149, 52.1086) centre (24.3817, 52.1086) ccw
  line L417 (25.2149, 52.1086) -> (25.2149, 79.6873)
  arc A44 (25.2149, 79.6873) -> (24.3817, 80.5205) centre (24.3817, 79.6873) ccw
  line L418 (24.3817, 80.5205) -> (1.238, 80.5205)
  line L419 (1.238, 80.5205) -> (1.238, 81.354)
  line L420 (1.238, 81.354) -> (24.3817, 81.354)
  arc A45 (26.0484, 79.6873) -> (24.3817, 81.354) centre (24.3817, 79.6873) ccw
  line L421 (26.0484, 79.6873) -> (26.0484, 52.1086)
  arc A46 (24.3817, 50.4419) -> (26.0484, 52.1086) centre (24.3817, 52.1086) ccw
  line L422 (24.3817, 50.4419) -> (-22.8357, 50.4419)
  arc A47 (-24.5023, 52.1086) -> (-22.8357, 50.4419) centre (-22.8357, 52.1086) ccw
  line L423 (-24.5023, 52.1086) -> (-24.5023, 79.6873)
  arc A48 (-20.3376, 42.1374) -> (-22.0042, 40.4707) centre (-20.3376, 40.4707) ccw
  line L424 (-20.3376, 42.1374) -> (-19.6993, 42.1374)
  line L425 (-19.6993, 42.1374) -> (-19.6993, 41.2955)
  line L426 (-19.6993, 41.2955) -> (-20.3376, 41.2955)
  arc A49 (-20.3376, 41.2955) -> (-21.1624, 40.4707) centre (-20.3376, 40.4707) ccw
  line L427 (-21.1624, 40.4707) -> (-21.1624, 10.7293)
  arc A50 (-21.1624, 10.7293) -> (-20.3376, 9.9045) centre (-20.3376, 10.7293) ccw
  line L428 (-20.3376, 9.9045) -> (21.9158, 9.9045)
  arc A51 (21.9158, 9.9045) -> (22.7406, 10.7293) centre (21.9158, 10.7293) ccw
  line L429 (22.7406, 10.7293) -> (22.7406, 40.4707)
  arc A52 (22.7406, 40.4707) -> (21.9158, 41.2955) centre (21.9158, 40.4707) ccw
  line L430 (21.9158, 41.2955) -> (-10.9584, 41.2955)
  line L431 (-10.9584, 41.2955) -> (-10.9584, 42.1374)
  line L432 (-10.9584, 42.1374) -> (21.9158, 42.1374)
  arc A53 (23.5825, 40.4707) -> (21.9158, 42.1374) centre (21.9158, 40.4707) ccw
  line L433 (23.5825, 40.4707) -> (23.5825, 10.7293)
  arc A54 (21.9158, 9.0626) -> (23.5825, 10.7293) centre (21.9158, 10.7293) ccw
  line L434 (21.9158, 9.0626) -> (-20.3376, 9.0626)
  arc A55 (-22.0042, 10.7293) -> (-20.3376, 9.0626) centre (-20.3376, 10.7293) ccw
  line L435 (-22.0042, 10.7293) -> (-22.0042, 40.4707)
  line L436 (-19.6367, 6.3555) -> (-19.6367, 5.5222)
  line L437 (-19.6367, 5.5222) -> (-20.3351, 5.5222)
  arc A56 (-20.3351, 5.5222) -> (-21.1685, 4.6888) centre (-20.3351, 4.6888) ccw
  line L438 (-21.1685, 4.6888) -> (-21.1685, -14.4814)
  arc A57 (-21.1685, -14.4814) -> (-20.3351, -15.3147) centre (-20.3351, -14.4814) ccw
  line L439 (-20.3351, -15.3147) -> (21.8817, -15.3147)
  arc A58 (21.8817, -15.3147) -> (22.715, -14.4814) centre (21.8817, -14.4814) ccw
  line L440 (22.715, -14.4814) -> (22.715, 4.6888)
  arc A59 (22.715, 4.6888) -> (21.8817, 5.5222) centre (21.8817, 4.6888) ccw
  line L441 (21.8817, 5.5222) -> (-12.2369, 5.5222)
  line L442 (-12.2369, 5.5222) -> (-12.2369, 6.3555)
  line L443 (-12.2369, 6.3555) -> (21.8817, 6.3555)
  arc A60 (23.5483, 4.6888) -> (21.8817, 6.3555) centre (21.8817, 4.6888) ccw
  line L444 (23.5483, 4.6888) -> (23.5483, -14.4814)
  arc A61 (21.8817, -16.148) -> (23.5483, -14.4814) centre (21.8817, -14.4814) ccw
  line L445 (21.8817, -16.148) -> (-20.3351, -16.148)
  arc A62 (-22.0018, -14.4814) -> (-20.3351, -16.148) centre (-20.3351, -14.4814) ccw
  line L446 (-22.0018, -14.4814) -> (-22.0018, 4.6888)
  arc A63 (-20.3351, 6.3555) -> (-22.0018, 4.6888) centre (-20.3351, 4.6888) ccw
  line L447 (-20.3351, 6.3555) -> (-19.6367, 6.3555)
  line L448 (-14.0455, 46.8954) -> (-13.2163, 46.8954)
  line L449 (-13.2163, 46.8954) -> (-13.2163, 47.7246)
  line L450 (-13.2163, 47.7246) -> (-14.0455, 47.7246)
  line L451 (-13.2163, 45.4417) -> (-13.2163, 46.4791)
  line L452 (-13.2163, 46.4791) -> (-13.7263, 46.4791)
  line L453 (-13.7263, 46.4791) -> (-14.493, 45.3273)
  line L454 (1.4715, -46.542) -> (1.4715, -58.6253)
  line L455 (1.4715, -58.6253) -> (20.6382, -58.6253)
  line L456 (20.6382, -58.6253) -> (20.6382, -46.542)
  line L457 (20.6382, -46.542) -> (1.4715, -46.542)
  line L458 (0.2491, 39.713) -> (0.2491, 27.6296)
  line L459 (0.2491, 27.6296) -> (19.4158, 27.6296)
  line L460 (19.4158, 27.6296) -> (19.4158, 39.713)
  line L461 (19.4158, 39.713) -> (0.2491, 39.713)
  arc A64 (26.6667, -92.9167) -> (29.1667, -90.4167) centre (26.6667, -90.4167) ccw
  line L462 (26.6667, -92.9167) -> (-26.6667, -92.9167)
  arc A65 (-29.1667, -90.4167) -> (-26.6667, -92.9167) centre (-26.6667, -90.4167) ccw
  line L463 (-29.1667, -90.4167) -> (-29.1667, 90.4167)
  arc A66 (-26.6667, 92.9167) -> (-29.1667, 90.4167) centre (-26.6667, 90.4167) ccw
  line L464 (-26.6667, 92.9167) -> (26.6667, 92.9167)
  arc A67 (29.1667, 90.4167) -> (26.6667, 92.9167) centre (26.6667, 90.4167) ccw
  line L465 (29.1667, 90.4167) -> (29.1667, -90.4167)
  spline S0 degree 2 poles (19.5149, -63.8455) (19.3067, -63.8455) (19.3067, -63.6373) knots 0 0 0 1 1 1
  line L466 (19.5149, -63.8455) -> (19.3067, -63.8455) construction
  line L467 (19.3067, -63.8455) -> (19.3067, -63.6373) construction
  spline S1 degree 2 poles (18.0508, -63.7032) (18.0057, -63.8455) (17.867, -63.8455) knots 0 0 0 1 1 1
  line L468 (18.0508, -63.7032) -> (18.0057, -63.8455) construction
  line L469 (18.0057, -63.8455) -> (17.867, -63.8455) construction
  spline S2 degree 2 poles (17.867, -63.8455) (17.6484, -63.8455) (17.6484, -63.6477) knots 0 0 0 1 1 1
  line L470 (17.867, -63.8455) -> (17.6484, -63.8455) construction
  line L471 (17.6484, -63.8455) -> (17.6484, -63.6477) construction
  spline S3 degree 2 poles (17.6484, -63.6477) (17.6484, -63.6096) (17.6623, -63.5714) knots 0 0 0 1 1 1
  line L472 (17.6484, -63.6477) -> (17.6484, -63.6096) construction
  line L473 (17.6484, -63.6096) -> (17.6623, -63.5714) construction
  line L474 (17.6623, -63.5714) -> (18.4845, -61.0804)
  spline S4 degree 2 poles (18.4845, -61.0804) (18.5296, -60.9382) (18.6788, -60.9382) knots 0 0 0 1 1 1
  line L475 (18.4845, -61.0804) -> (18.5296, -60.9382) construction
  line L476 (18.5296, -60.9382) -> (18.6788, -60.9382) construction
  line L477 (18.6788, -60.9382) -> (19.5149, -60.9382)
  spline S5 degree 2 poles (19.5149, -60.9382) (19.7231, -60.9382) (19.7231, -61.1463) knots 0 0 0 1 1 1
  line L478 (19.5149, -60.9382) -> (19.7231, -60.9382) construction
  line L479 (19.7231, -60.9382) -> (19.7231, -61.1463) construction
  line L480 (19.7231, -61.1463) -> (19.7231, -63.6373)
  spline S6 degree 2 poles (19.7231, -63.6373) (19.7231, -63.8455) (19.5149, -63.8455) knots 0 0 0 1 1 1
  line L481 (19.7231, -63.6373) -> (19.7231, -63.8455) construction
  line L482 (19.7231, -63.8455) -> (19.5149, -63.8455) construction
  spline S7 degree 2 poles (7.8857, -63.8455) (7.6775, -63.8455) (7.6775, -63.6373) knots 0 0 0 1 1 1
  line L483 (7.8857, -63.8455) -> (7.6775, -63.8455) construction
  line L484 (7.6775, -63.8455) -> (7.6775, -63.6373) construction
  line L485 (7.6775, -63.6373) -> (7.6775, -61.7708)
  spline S8 degree 2 poles (7.6775, -61.7708) (7.6775, -61.6008) (7.4347, -61.3545) (7.2647, -61.3545) knots 0 0 0 1 2 2 2
  line L486 (7.6775, -61.7708) -> (7.6775, -61.6008) construction
  line L487 (7.6775, -61.6008) -> (7.4347, -61.3545) construction
  line L488 (7.4347, -61.3545) -> (7.2647, -61.3545) construction
  spline S9 degree 2 poles (6.4355, -63.6373) (6.4355, -63.8455) (6.2274, -63.8455) knots 0 0 0 1 1 1
  line L489 (6.4355, -63.6373) -> (6.4355, -63.8455) construction
  line L490 (6.4355, -63.8455) -> (6.2274, -63.8455) construction
  spline S10 degree 2 poles (6.2274, -63.8455) (6.0192, -63.8455) (6.0192, -63.6373) knots 0 0 0 1 1 1
  line L491 (6.2274, -63.8455) -> (6.0192, -63.8455) construction
  line L492 (6.0192, -63.8455) -> (6.0192, -63.6373) construction
  line L493 (6.0192, -63.6373) -> (6.0192, -61.1463)
  spline S11 degree 2 poles (6.0192, -61.1463) (6.0192, -60.9382) (6.2274, -60.9382) knots 0 0 0 1 1 1
  line L494 (6.0192, -61.1463) -> (6.0192, -60.9382) construction
  line L495 (6.0192, -60.9382) -> (6.2274, -60.9382) construction
  line L496 (6.2274, -60.9382) -> (7.2647, -60.9382)
  spline S12 degree 2 poles (7.2647, -60.9382) (7.6082, -60.9382) (8.0939, -61.4239) (8.0939, -61.7674) knots 0 0 0 1 2 2 2
  line L497 (7.2647, -60.9382) -> (7.6082, -60.9382) construction
  line L498 (7.6082, -60.9382) -> (8.0939, -61.4239) construction
  line L499 (8.0939, -61.4239) -> (8.0939, -61.7674) construction
  line L500 (8.0939, -61.7674) -> (8.0939, -63.6373)
  spline S13 degree 2 poles (8.0939, -63.6373) (8.0939, -63.8455) (7.8857, -63.8455) knots 0 0 0 1 1 1
  line L501 (8.0939, -63.6373) -> (8.0939, -63.8455) construction
  line L502 (8.0939, -63.8455) -> (7.8857, -63.8455) construction
  spline S14 degree 2 poles (4.3574, -63.4292) (4.5274, -63.4292) (4.7702, -63.1828) (4.7702, -63.0128) knots 0 0 0 1 2 2 2
  line L503 (4.3574, -63.4292) -> (4.5274, -63.4292) construction
  line L504 (4.5274, -63.4292) -> (4.7702, -63.1828) construction
  line L505 (4.7702, -63.1828) -> (4.7702, -63.0128) construction
  spline S15 degree 2 poles (3.9411, -61.3545) (3.7711, -61.3545) (3.5282, -61.6008) (3.5282, -61.7708) knots 0 0 0 1 2 2 2
  line L506 (3.9411, -61.3545) -> (3.7711, -61.3545) construction
  line L507 (3.7711, -61.3545) -> (3.5282, -61.6008) construction
  line L508 (3.5282, -61.6008) -> (3.5282, -61.7708) construction
  line L509 (3.5282, -61.7708) -> (3.5282, -63.0128)
  spline S16 degree 2 poles (3.5282, -63.0128) (3.5282, -63.1828) (3.7711, -63.4292) (3.9411, -63.4292) knots 0 0 0 1 2 2 2
  line L510 (3.5282, -63.0128) -> (3.5282, -63.1828) construction
  line L511 (3.5282, -63.1828) -> (3.7711, -63.4292) construction
  line L512 (3.7711, -63.4292) -> (3.9411, -63.4292) construction
  line L513 (3.9411, -63.4292) -> (4.3574, -63.4292)
  line L514 (4.3574, -63.8455) -> (3.9411, -63.8455)
  spline S17 degree 2 poles (3.9411, -63.8455) (3.6011, -63.8455) (3.1119, -63.3598) (3.1119, -63.0163) knots 0 0 0 1 2 2 2
  line L515 (3.9411, -63.8455) -> (3.6011, -63.8455) construction
  line L516 (3.6011, -63.8455) -> (3.1119, -63.3598) construction
  line L517 (3.1119, -63.3598) -> (3.1119, -63.0163) construction
  line L518 (3.1119, -63.0163) -> (3.1119, -61.7674)
  spline S18 degree 2 poles (3.1119, -61.7674) (3.1119, -61.4239) (3.6011, -60.9382) (3.9411, -60.9382) knots 0 0 0 1 2 2 2
  line L519 (3.1119, -61.7674) -> (3.1119, -61.4239) construction
  line L520 (3.1119, -61.4239) -> (3.6011, -60.9382) construction
  line L521 (3.6011, -60.9382) -> (3.9411, -60.9382) construction
  line L522 (3.9411, -60.9382) -> (4.9784, -60.9382)
  spline S19 degree 2 poles (4.9784, -60.9382) (5.1866, -60.9382) (5.1866, -61.1463) knots 0 0 0 1 1 1
  line L523 (4.9784, -60.9382) -> (5.1866, -60.9382) construction
  line L524 (5.1866, -60.9382) -> (5.1866, -61.1463) construction
  line L525 (5.1866, -61.1463) -> (5.1866, -63.0094)
  spline S20 degree 2 poles (5.1866, -63.0094) (5.1866, -63.3216) (5.478, -63.4465) knots 0 0 0 1 1 1
  line L526 (5.1866, -63.0094) -> (5.1866, -63.3216) construction
  line L527 (5.1866, -63.3216) -> (5.478, -63.4465) construction
  spline S21 degree 2 poles (5.478, -63.4465) (5.6064, -63.4985) (5.6064, -63.6304) knots 0 0 0 1 1 1
  line L528 (5.478, -63.4465) -> (5.6064, -63.4985) construction
  line L529 (5.6064, -63.4985) -> (5.6064, -63.6304) construction
  spline S22 degree 2 poles (5.6064, -63.6304) (5.6064, -63.7171) (5.4884, -63.849) (5.4017, -63.849) knots 0 0 0 1 2 2 2
  line L530 (5.6064, -63.6304) -> (5.6064, -63.7171) construction
  line L531 (5.6064, -63.7171) -> (5.4884, -63.849) construction
  line L532 (5.4884, -63.849) -> (5.4017, -63.849) construction
  spline S23 degree 2 poles (5.4017, -63.849) (5.3566, -63.849) (5.3115, -63.8281) knots 0 0 0 1 1 1
  line L533 (5.4017, -63.849) -> (5.3566, -63.849) construction
  line L534 (5.3566, -63.849) -> (5.3115, -63.8281) construction
  spline S24 degree 2 poles (5.3115, -63.8281) (5.1033, -63.7379) (4.9749, -63.5714) knots 0 0 0 1 1 1
  line L535 (5.3115, -63.8281) -> (5.1033, -63.7379) construction
  line L536 (5.1033, -63.7379) -> (4.9749, -63.5714) construction
  spline S25 degree 2 poles (4.9749, -63.5714) (4.7251, -63.8455) (4.3574, -63.8455) knots 0 0 0 1 1 1
  line L537 (4.9749, -63.5714) -> (4.7251, -63.8455) construction
  line L538 (4.7251, -63.8455) -> (4.3574, -63.8455) construction
  spline S26 degree 2 poles (-3.5353, -61.1463) (-3.5353, -60.9382) (-3.3272, -60.9382) knots 0 0 0 1 1 1
  line L539 (-3.5353, -61.1463) -> (-3.5353, -60.9382) construction
  line L540 (-3.5353, -60.9382) -> (-3.3272, -60.9382) construction
  spline S27 degree 2 poles (-3.3272, -60.9382) (-3.119, -60.9382) (-3.119, -61.1463) knots 0 0 0 1 1 1
  line L541 (-3.3272, -60.9382) -> (-3.119, -60.9382) construction
  line L542 (-3.119, -60.9382) -> (-3.119, -61.1463) construction
  line L543 (-3.119, -61.1463) -> (-3.119, -63.6373)
  spline S28 degree 2 poles (-3.119, -63.6373) (-3.119, -63.8455) (-3.3272, -63.8455) knots 0 0 0 1 1 1
  line L544 (-3.119, -63.6373) -> (-3.119, -63.8455) construction
  line L545 (-3.119, -63.8455) -> (-3.3272, -63.8455) construction
  spline S29 degree 2 poles (-3.3272, -63.8455) (-3.5353, -63.8455) (-3.5353, -63.6373) knots 0 0 0 1 1 1
  line L546 (-3.3272, -63.8455) -> (-3.5353, -63.8455) construction
  line L547 (-3.5353, -63.8455) -> (-3.5353, -63.6373) construction
  spline S30 degree 2 poles (-4.7774, -63.6373) (-4.7774, -63.8455) (-4.9855, -63.8455) knots 0 0 0 1 1 1
  line L548 (-4.7774, -63.6373) -> (-4.7774, -63.8455) construction
  line L549 (-4.7774, -63.8455) -> (-4.9855, -63.8455) construction
  spline S31 degree 2 poles (-4.9855, -63.8455) (-5.1937, -63.8455) (-5.1937, -63.6373) knots 0 0 0 1 1 1
  line L550 (-4.9855, -63.8455) -> (-5.1937, -63.8455) construction
  line L551 (-5.1937, -63.8455) -> (-5.1937, -63.6373) construction
  line L552 (-5.1937, -63.6373) -> (-5.1937, -61.1463)
  spline S32 degree 2 poles (-5.1937, -61.1463) (-5.1937, -60.9382) (-4.9855, -60.9382) knots 0 0 0 1 1 1
  line L553 (-5.1937, -61.1463) -> (-5.1937, -60.9382) construction
  line L554 (-5.1937, -60.9382) -> (-4.9855, -60.9382) construction
  spline S33 degree 2 poles (-4.9855, -60.9382) (-4.7774, -60.9382) (-4.7774, -61.1463) knots 0 0 0 1 1 1
  line L555 (-4.9855, -60.9382) -> (-4.7774, -60.9382) construction
  line L556 (-4.7774, -60.9382) -> (-4.7774, -61.1463) construction
  spline S34 degree 2 poles (-6.9387, -63.4292) (-6.7375, -63.4292) (-6.4426, -63.1377) (-6.4426, -62.9296) knots 0 0 0 1 2 2 2
  line L557 (-6.9387, -63.4292) -> (-6.7375, -63.4292) construction
  line L558 (-6.7375, -63.4292) -> (-6.4426, -63.1377) construction
  line L559 (-6.4426, -63.1377) -> (-6.4426, -62.9296) construction
  line L560 (-6.4426, -62.9296) -> (-6.4426, -61.8541)
  spline S35 degree 2 poles (-6.4426, -61.8541) (-6.4426, -61.6494) (-6.7375, -61.3545) (-6.9387, -61.3545) knots 0 0 0 1 2 2 2
  line L561 (-6.4426, -61.8541) -> (-6.4426, -61.6494) construction
  line L562 (-6.4426, -61.6494) -> (-6.7375, -61.3545) construction
  line L563 (-6.7375, -61.3545) -> (-6.9387, -61.3545) construction
  line L564 (-6.9387, -61.3545) -> (-7.1885, -61.3545)
  spline S36 degree 2 poles (-7.1885, -61.3545) (-7.3932, -61.3545) (-7.6847, -61.6494) (-7.6847, -61.8541) knots 0 0 0 1 2 2 2
  line L565 (-7.1885, -61.3545) -> (-7.3932, -61.3545) construction
  line L566 (-7.3932, -61.3545) -> (-7.6847, -61.6494) construction
  line L567 (-7.6847, -61.6494) -> (-7.6847, -61.8541) construction
  line L568 (-7.6847, -61.8541) -> (-7.6847, -62.9296)
  spline S37 degree 2 poles (-7.6847, -62.9296) (-7.6847, -63.1377) (-7.3932, -63.4292) (-7.1885, -63.4292) knots 0 0 0 1 2 2 2
  line L569 (-7.6847, -62.9296) -> (-7.6847, -63.1377) construction
  line L570 (-7.6847, -63.1377) -> (-7.3932, -63.4292) construction
  line L571 (-7.3932, -63.4292) -> (-7.1885, -63.4292) construction
  line L572 (-7.1885, -63.4292) -> (-6.9387, -63.4292)
  line L573 (-6.9387, -63.8455) -> (-7.1885, -63.8455)
  spline S38 degree 2 poles (-7.1885, -63.8455) (-7.5632, -63.8455) (-8.101, -63.3112) (-8.101, -62.933) knots 0 0 0 1 2 2 2
  line L574 (-7.1885, -63.8455) -> (-7.5632, -63.8455) construction
  line L575 (-7.5632, -63.8455) -> (-8.101, -63.3112) construction
  line L576 (-8.101, -63.3112) -> (-8.101, -62.933) construction
  line L577 (-8.101, -62.933) -> (-8.101, -61.8506)
  spline S39 degree 2 poles (-8.101, -61.8506) (-8.101, -61.4725) (-7.5632, -60.9382) (-7.1885, -60.9382) knots 0 0 0 1 2 2 2
  line L578 (-8.101, -61.8506) -> (-8.101, -61.4725) construction
  line L579 (-8.101, -61.4725) -> (-7.5632, -60.9382) construction
  line L580 (-7.5632, -60.9382) -> (-7.1885, -60.9382) construction
  line L581 (-7.1885, -60.9382) -> (-6.9387, -60.9382)
  spline S40 degree 2 poles (-6.9387, -60.9382) (-6.5606, -60.9382) (-6.0263, -61.4725) (-6.0263, -61.8506) knots 0 0 0 1 2 2 2
  line L582 (-6.9387, -60.9382) -> (-6.5606, -60.9382) construction
  line L583 (-6.5606, -60.9382) -> (-6.0263, -61.4725) construction
  line L584 (-6.0263, -61.4725) -> (-6.0263, -61.8506) construction
  line L585 (-6.0263, -61.8506) -> (-6.0263, -62.933)
  spline S41 degree 2 poles (-6.0263, -62.933) (-6.0263, -63.3147) (-6.5606, -63.8455) (-6.9387, -63.8455) knots 0 0 0 1 2 2 2
  line L586 (-6.0263, -62.933) -> (-6.0263, -63.3147) construction
  line L587 (-6.0263, -63.3147) -> (-6.5606, -63.8455) construction
  line L588 (-6.5606, -63.8455) -> (-6.9387, -63.8455) construction
  line L589 (-13.5409, -62.9747) -> (-13.5409, -63.6373)
  spline S42 degree 2 poles (-13.5409, -63.6373) (-13.5409, -63.8455) (-13.749, -63.8455) knots 0 0 0 1 1 1
  line L590 (-13.5409, -63.6373) -> (-13.5409, -63.8455) construction
  line L591 (-13.5409, -63.8455) -> (-13.749, -63.8455) construction
  spline S43 degree 2 poles (-13.749, -63.8455) (-13.9572, -63.8455) (-13.9572, -63.6373) knots 0 0 0 1 1 1
  line L592 (-13.749, -63.8455) -> (-13.9572, -63.8455) construction
  line L593 (-13.9572, -63.8455) -> (-13.9572, -63.6373) construction
  line L594 (-13.9572, -63.6373) -> (-13.9572, -61.1463)
  spline S44 degree 2 poles (-13.9572, -61.1463) (-13.9572, -60.9382) (-13.749, -60.9382) knots 0 0 0 1 1 1
  line L595 (-13.9572, -61.1463) -> (-13.9572, -60.9382) construction
  line L596 (-13.9572, -60.9382) -> (-13.749, -60.9382) construction
  spline S45 degree 2 poles (-13.749, -60.9382) (-13.5409, -60.9382) (-13.5409, -61.1463) knots 0 0 0 1 1 1
  line L597 (-13.749, -60.9382) -> (-13.5409, -60.9382) construction
  line L598 (-13.5409, -60.9382) -> (-13.5409, -61.1463) construction
  spline S46 degree 2 poles (-12.2225, -60.9868) (-12.167, -60.9243) (-12.0907, -60.9243) knots 0 0 0 1 1 1
  line L599 (-12.2225, -60.9868) -> (-12.167, -60.9243) construction
  line L600 (-12.167, -60.9243) -> (-12.0907, -60.9243) construction
  spline S47 degree 2 poles (-12.0907, -60.9243) (-12.0074, -60.9243) (-11.8825, -61.0596) (-11.8825, -61.1498) knots 0 0 0 1 2 2 2
  line L601 (-12.0907, -60.9243) -> (-12.0074, -60.9243) construction
  line L602 (-12.0074, -60.9243) -> (-11.8825, -61.0596) construction
  line L603 (-11.8825, -61.0596) -> (-11.8825, -61.1498) construction
  spline S48 degree 2 poles (-11.8825, -61.1498) (-11.8825, -61.2365) (-11.9485, -61.3025) knots 0 0 0 1 1 1
  line L604 (-11.8825, -61.1498) -> (-11.8825, -61.2365) construction
  line L605 (-11.8825, -61.2365) -> (-11.9485, -61.3025) construction
  spline S49 degree 2 poles (-11.9276, -63.502) (-11.8825, -63.5714) (-11.8825, -63.6408) knots 0 0 0 1 1 1
  line L606 (-11.9276, -63.502) -> (-11.8825, -63.5714) construction
  line L607 (-11.8825, -63.5714) -> (-11.8825, -63.6408) construction
  spline S50 degree 2 poles (-11.8825, -63.6408) (-11.8825, -63.7275) (-12.0178, -63.8524) (-12.0942, -63.8524) knots 0 0 0 1 2 2 2
  line L608 (-11.8825, -63.6408) -> (-11.8825, -63.7275) construction
  line L609 (-11.8825, -63.7275) -> (-12.0178, -63.8524) construction
  line L610 (-12.0178, -63.8524) -> (-12.0942, -63.8524) construction
  spline S51 degree 2 poles (-12.0942, -63.8524) (-12.1913, -63.8524) (-12.2434, -63.7692) knots 0 0 0 1 1 1
  line L611 (-12.0942, -63.8524) -> (-12.1913, -63.8524) construction
  line L612 (-12.1913, -63.8524) -> (-12.2434, -63.7692) construction
  line L613 (-12.2434, -63.7692) -> (-13.076, -62.4855)
  spline S52 degree 2 poles (-13.076, -62.4855) (-13.2009, -62.6173) (-13.5409, -62.9747) knots 0 0 0 1 1 1
  line L614 (-13.076, -62.4855) -> (-13.2009, -62.6173) construction
  line L615 (-13.2009, -62.6173) -> (-13.5409, -62.9747) construction
  spline S53 degree 2 poles (-15.5774, -63.4292) (-15.4074, -63.4292) (-15.1645, -63.1828) (-15.1645, -63.0128) knots 0 0 0 1 2 2 2
  line L616 (-15.5774, -63.4292) -> (-15.4074, -63.4292) construction
  line L617 (-15.4074, -63.4292) -> (-15.1645, -63.1828) construction
  line L618 (-15.1645, -63.1828) -> (-15.1645, -63.0128) construction
  spline S54 degree 2 poles (-15.9937, -61.3545) (-16.1637, -61.3545) (-16.4066, -61.6008) (-16.4066, -61.7708) knots 0 0 0 1 2 2 2
  line L619 (-15.9937, -61.3545) -> (-16.1637, -61.3545) construction
  line L620 (-16.1637, -61.3545) -> (-16.4066, -61.6008) construction
  line L621 (-16.4066, -61.6008) -> (-16.4066, -61.7708) construction
  line L622 (-16.4066, -61.7708) -> (-16.4066, -63.0128)
  spline S55 degree 2 poles (-16.4066, -63.0128) (-16.4066, -63.1828) (-16.1637, -63.4292) (-15.9937, -63.4292) knots 0 0 0 1 2 2 2
  line L623 (-16.4066, -63.0128) -> (-16.4066, -63.1828) construction
  line L624 (-16.4066, -63.1828) -> (-16.1637, -63.4292) construction
  line L625 (-16.1637, -63.4292) -> (-15.9937, -63.4292) construction
  line L626 (-15.9937, -63.4292) -> (-15.5774, -63.4292)
  line L627 (-15.5774, -63.8455) -> (-15.9937, -63.8455)
  spline S56 degree 2 poles (-15.9937, -63.8455) (-16.3337, -63.8455) (-16.8229, -63.3598) (-16.8229, -63.0163) knots 0 0 0 1 2 2 2
  line L628 (-15.9937, -63.8455) -> (-16.3337, -63.8455) construction
  line L629 (-16.3337, -63.8455) -> (-16.8229, -63.3598) construction
  line L630 (-16.8229, -63.3598) -> (-16.8229, -63.0163) construction
  line L631 (-16.8229, -63.0163) -> (-16.8229, -61.7674)
  spline S57 degree 2 poles (-16.8229, -61.7674) (-16.8229, -61.4239) (-16.3337, -60.9382) (-15.9937, -60.9382) knots 0 0 0 1 2 2 2
  line L632 (-16.8229, -61.7674) -> (-16.8229, -61.4239) construction
  line L633 (-16.8229, -61.4239) -> (-16.3337, -60.9382) construction
  line L634 (-16.3337, -60.9382) -> (-15.9937, -60.9382) construction
  line L635 (-15.9937, -60.9382) -> (-14.9564, -60.9382)
  spline S58 degree 2 poles (-14.9564, -60.9382) (-14.7482, -60.9382) (-14.7482, -61.1463) knots 0 0 0 1 1 1
  line L636 (-14.9564, -60.9382) -> (-14.7482, -60.9382) construction
  line L637 (-14.7482, -60.9382) -> (-14.7482, -61.1463) construction
  line L638 (-14.7482, -61.1463) -> (-14.7482, -63.0094)
  spline S59 degree 2 poles (-14.7482, -63.0094) (-14.7482, -63.3216) (-14.4568, -63.4465) knots 0 0 0 1 1 1
  line L639 (-14.7482, -63.0094) -> (-14.7482, -63.3216) construction
  line L640 (-14.7482, -63.3216) -> (-14.4568, -63.4465) construction
  spline S60 degree 2 poles (-14.4568, -63.4465) (-14.3284, -63.4985) (-14.3284, -63.6304) knots 0 0 0 1 1 1
  line L641 (-14.4568, -63.4465) -> (-14.3284, -63.4985) construction
  line L642 (-14.3284, -63.4985) -> (-14.3284, -63.6304) construction
  spline S61 degree 2 poles (-14.3284, -63.6304) (-14.3284, -63.7171) (-14.4464, -63.849) (-14.5331, -63.849) knots 0 0 0 1 2 2 2
  line L643 (-14.3284, -63.6304) -> (-14.3284, -63.7171) construction
  line L644 (-14.3284, -63.7171) -> (-14.4464, -63.849) construction